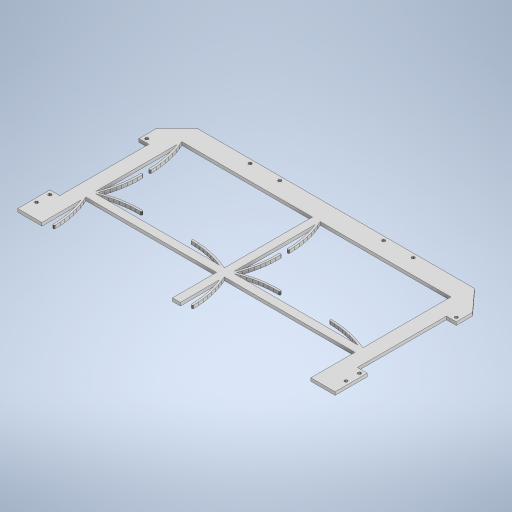
# Autodesk Inventor part: deck_top
Saved by Autodesk Inventor 2024.1 (Build 281209000, 209)
## iProperties
Created: 2024-06-24
Part Number: deck_top
Material: Generic
Document SubType Name: Modeling
Designer: pab2
Density: 1 g/cm^3
Appearance: Default
Author: pab2
Autodesk Inventor part; units mm, degrees
ref_plane "YZ Plane" through (0, 0, 0) normal (1, 0, 0) x (0, 1, 0)
ref_plane "XZ Plane" through (0, 0, 0) normal (0, 1, 0) x (-1, 0, 0)
ref_plane "XY Plane" through (0, 0, 0) normal (0, 0, 1) x (1, 0, 0)
sketch "Sketch1" plane through (0, 0, 0) normal (0, 1, 0) x (-1, 0, 0)
  line L0 (377.2253, 565.1147) -> (377.7897, 565.2558)
  line L1 (377.7897, 565.2558) -> (378.2836, 565.5733)
  line L2 (378.2836, 565.5733) -> (378.6011, 566.0672)
  line L3 (378.6011, 566.0672) -> (378.7422, 566.6316)
  line L4 (378.7422, 566.6316) -> (378.6011, 567.1961)
  line L5 (378.6011, 567.1961) -> (378.2836, 567.69)
  line L6 (378.2836, 567.69) -> (377.7897, 568.0075)
  line L7 (377.7897, 568.0075) -> (377.2253, 568.1133)
  line L8 (377.2253, 568.1133) -> (376.6608, 568.0075)
  line L9 (376.6608, 568.0075) -> (376.167, 567.69)
  line L10 (376.167, 567.69) -> (375.8495, 567.1961)
  line L11 (375.8495, 567.1961) -> (375.7436, 566.6316)
  line L12 (375.7436, 566.6316) -> (375.8495, 566.0672)
  line L13 (375.8495, 566.0672) -> (376.167, 565.5733)
  line L14 (376.167, 565.5733) -> (376.6608, 565.2558)
  line L15 (376.6608, 565.2558) -> (377.2253, 565.1147)
  line L16 (347.2392, 565.1147) -> (347.8036, 565.2558)
  line L17 (347.8036, 565.2558) -> (348.2975, 565.5733)
  line L18 (348.2975, 565.5733) -> (348.615, 566.0672)
  line L19 (348.615, 566.0672) -> (348.7208, 566.6316)
  line L20 (348.7208, 566.6316) -> (348.615, 567.1961)
  line L21 (348.615, 567.1961) -> (348.2975, 567.69)
  line L22 (348.2975, 567.69) -> (347.8036, 568.0075)
  line L23 (347.8036, 568.0075) -> (347.2392, 568.1133)
  line L24 (347.2392, 568.1133) -> (346.6395, 568.0075)
  line L25 (346.6395, 568.0075) -> (346.1809, 567.69)
  line L26 (346.1809, 567.69) -> (345.8281, 567.1961)
  line L27 (345.8281, 567.1961) -> (345.7222, 566.6316)
  line L28 (345.7222, 566.6316) -> (345.8281, 566.0672)
  line L29 (345.8281, 566.0672) -> (346.1809, 565.5733)
  line L30 (346.1809, 565.5733) -> (346.6395, 565.2558)
  line L31 (346.6395, 565.2558) -> (347.2392, 565.1147)
  line L32 (212.2311, 565.1147) -> (212.7956, 565.2558)
  line L33 (212.7956, 565.2558) -> (213.2895, 565.5733)
  line L34 (213.2895, 565.5733) -> (213.607, 566.0672)
  line L35 (213.607, 566.0672) -> (213.7128, 566.6316)
  line L36 (213.7128, 566.6316) -> (213.607, 567.1961)
  line L37 (213.607, 567.1961) -> (213.2895, 567.69)
  line L38 (213.2895, 567.69) -> (212.7956, 568.0075)
  line L39 (212.7956, 568.0075) -> (212.2311, 568.1133)
  line L40 (212.2311, 568.1133) -> (211.6667, 568.0075)
  line L41 (211.6667, 568.0075) -> (211.1728, 567.69)
  line L42 (211.1728, 567.69) -> (210.8553, 567.1961)
  line L43 (210.8553, 567.1961) -> (210.7142, 566.6316)
  line L44 (210.7142, 566.6316) -> (210.8553, 566.0672)
  line L45 (210.8553, 566.0672) -> (211.1728, 565.5733)
  line L46 (211.1728, 565.5733) -> (211.6667, 565.2558)
  line L47 (211.6667, 565.2558) -> (212.2311, 565.1147)
  line L48 (423.7214, 631.1547) -> (423.792, 635.9878)
  line L49 (423.792, 635.9878) -> (424.1094, 640.8208)
  line L50 (424.1094, 640.8208) -> (424.6386, 645.6186)
  line L51 (424.6386, 645.6186) -> (425.3795, 650.4164)
  line L52 (425.3795, 650.4164) -> (426.4025, 655.1436)
  line L53 (426.4025, 655.1436) -> (427.6019, 659.8356)
  line L54 (427.6019, 659.8356) -> (429.0483, 664.4569)
  line L55 (429.0483, 664.4569) -> (430.7417, 668.9725)
  line L56 (421.7106, 631.1194) -> (421.8164, 630.7314)
  line L57 (421.8164, 630.7314) -> (422.0281, 630.4139)
  line L58 (422.0281, 630.4139) -> (422.3455, 630.2022)
  line L59 (422.3455, 630.2022) -> (422.7336, 630.1316)
  line L60 (422.7336, 630.1316) -> (423.1217, 630.2022)
  line L61 (423.1217, 630.2022) -> (423.4392, 630.4139)
  line L62 (423.4392, 630.4139) -> (423.6508, 630.7667)
  line L63 (423.6508, 630.7667) -> (423.7214, 631.1547)
  line L64 (428.5897, 668.9725) -> (426.9316, 664.4217)
  line L65 (426.9316, 664.4217) -> (425.5205, 659.8003)
  line L66 (425.5205, 659.8003) -> (424.3211, 655.1083)
  line L67 (424.3211, 655.1083) -> (423.3686, 650.3811)
  line L68 (423.3686, 650.3811) -> (422.5925, 645.5833)
  line L69 (422.5925, 645.5833) -> (422.0986, 640.7856)
  line L70 (422.0986, 640.7856) -> (421.7811, 635.9525)
  line L71 (421.7811, 635.9525) -> (421.7106, 631.1194)
  line L72 (390.7014, 662.1286) -> (395.5697, 662.1992)
  line L73 (395.5697, 662.1992) -> (400.3675, 662.4814)
  line L74 (400.3675, 662.4814) -> (405.2005, 663.0106)
  line L75 (405.2005, 663.0106) -> (409.963, 663.7514)
  line L76 (409.963, 663.7514) -> (414.7255, 664.7391)
  line L77 (414.7255, 664.7391) -> (419.4175, 665.9386)
  line L78 (419.4175, 665.9386) -> (424.0389, 667.3497)
  line L79 (424.0389, 667.3497) -> (428.5897, 668.9725)
  line L80 (390.7367, 664.1394) -> (390.3486, 664.0689)
  line L81 (390.3486, 664.0689) -> (390.0311, 663.8572)
  line L82 (390.0311, 663.8572) -> (389.8194, 663.5397)
  line L83 (389.8194, 663.5397) -> (389.7136, 663.1516)
  line L84 (389.7136, 663.1516) -> (389.7842, 662.7636)
  line L85 (389.7842, 662.7636) -> (389.9958, 662.4461)
  line L86 (389.9958, 662.4461) -> (390.3486, 662.1992)
  line L87 (390.3486, 662.1992) -> (390.7014, 662.1286)
  line L88 (428.5897, 671.1245) -> (424.0389, 669.4664)
  line L89 (424.0389, 669.4664) -> (419.4175, 668.02)
  line L90 (419.4175, 668.02) -> (414.7255, 666.7853)
  line L91 (414.7255, 666.7853) -> (409.9983, 665.7975)
  line L92 (409.9983, 665.7975) -> (405.2358, 665.0214)
  line L93 (405.2358, 665.0214) -> (400.4028, 664.4922)
  line L94 (400.4028, 664.4922) -> (395.5697, 664.21)
  line L95 (395.5697, 664.21) -> (390.7367, 664.1394)
  line L96 (428.5897, 671.1245) -> (303.8475, 671.1245)
  line L97 (338.7372, 664.1394) -> (334.2922, 664.3158)
  line L98 (334.2922, 664.3158) -> (329.812, 664.7039)
  line L99 (329.812, 664.7039) -> (325.4022, 665.2683)
  line L100 (325.4022, 665.2683) -> (320.9925, 666.0797)
  line L101 (320.9925, 666.0797) -> (316.6181, 667.0322)
  line L102 (316.6181, 667.0322) -> (312.3142, 668.2316)
  line L103 (312.3142, 668.2316) -> (308.0456, 669.5722)
  line L104 (308.0456, 669.5722) -> (303.8475, 671.1245)
  line L105 (338.702, 662.1286) -> (339.09, 662.1992)
  line L106 (339.09, 662.1992) -> (339.4075, 662.4108)
  line L107 (339.4075, 662.4108) -> (339.6545, 662.7283)
  line L108 (339.6545, 662.7283) -> (339.725, 663.1164)
  line L109 (339.725, 663.1164) -> (339.6545, 663.5044)
  line L110 (339.6545, 663.5044) -> (339.4428, 663.8219)
  line L111 (339.4428, 663.8219) -> (339.1253, 664.0336)
  line L112 (339.1253, 664.0336) -> (338.7372, 664.1394)
  line L113 (298.7322, 671.1245) -> (303.4947, 669.1136)
  line L114 (303.4947, 669.1136) -> (308.3278, 667.385)
  line L115 (308.3278, 667.385) -> (313.2667, 665.8681)
  line L116 (313.2667, 665.8681) -> (318.2761, 664.5981)
  line L117 (318.2761, 664.5981) -> (323.3208, 663.6103)
  line L118 (323.3208, 663.6103) -> (328.4361, 662.8342)
  line L119 (328.4361, 662.8342) -> (333.5514, 662.3755)
  line L120 (333.5514, 662.3755) -> (338.702, 662.1286)
  line L121 (298.7322, 671.1245) -> (298.7322, 582.1186)
  line L122 (298.7322, 582.1186) -> (430.7417, 582.1186)
  line L123 (421.7106, 622.1236) -> (421.9575, 616.9731)
  line L124 (421.9575, 616.9731) -> (422.4514, 611.8225)
  line L125 (422.4514, 611.8225) -> (423.1922, 606.7072)
  line L126 (423.1922, 606.7072) -> (424.2153, 601.6625)
  line L127 (424.2153, 601.6625) -> (425.45, 596.653)
  line L128 (425.45, 596.653) -> (426.967, 591.7141)
  line L129 (426.967, 591.7141) -> (428.7309, 586.8811)
  line L130 (428.7309, 586.8811) -> (430.7417, 582.1186)
  line L131 (423.7214, 622.1589) -> (423.6508, 622.5469)
  line L132 (423.6508, 622.5469) -> (423.4039, 622.8644)
  line L133 (423.4039, 622.8644) -> (423.0864, 623.0761)
  line L134 (423.0864, 623.0761) -> (422.6983, 623.1467)
  line L135 (422.6983, 623.1467) -> (422.3103, 623.0408)
  line L136 (422.3103, 623.0408) -> (421.9928, 622.8292)
  line L137 (421.9928, 622.8292) -> (421.7811, 622.5117)
  line L138 (421.7811, 622.5117) -> (421.7106, 622.1236)
  line L139 (430.7417, 587.2691) -> (429.1894, 591.4672)
  line L140 (429.1894, 591.4672) -> (427.8136, 595.7005)
  line L141 (427.8136, 595.7005) -> (426.6495, 600.0397)
  line L142 (426.6495, 600.0397) -> (425.6617, 604.3789)
  line L143 (425.6617, 604.3789) -> (424.8856, 608.7886)
  line L144 (424.8856, 608.7886) -> (424.2858, 613.2336)
  line L145 (424.2858, 613.2336) -> (423.8978, 617.6786)
  line L146 (423.8978, 617.6786) -> (423.7214, 622.1589)
  line L147 (430.7417, 587.2691) -> (430.7417, 668.9725)
  line L148 (281.7283, 622.1236) -> (281.94, 616.9731)
  line L149 (281.94, 616.9731) -> (282.4339, 611.8225)
  line L150 (282.4339, 611.8225) -> (283.21, 606.7072)
  line L151 (283.21, 606.7072) -> (284.1978, 601.6625)
  line L152 (284.1978, 601.6625) -> (285.4678, 596.653)
  line L153 (285.4678, 596.653) -> (286.9847, 591.7141)
  line L154 (286.9847, 591.7141) -> (288.7133, 586.8811)
  line L155 (288.7133, 586.8811) -> (290.7242, 582.1186)
  line L156 (283.7392, 622.1589) -> (283.6334, 622.5469)
  line L157 (283.6334, 622.5469) -> (283.4217, 622.8644)
  line L158 (283.4217, 622.8644) -> (283.1042, 623.0761)
  line L159 (283.1042, 623.0761) -> (282.7161, 623.1467)
  line L160 (282.7161, 623.1467) -> (282.3281, 623.0408)
  line L161 (282.3281, 623.0408) -> (282.0106, 622.8292)
  line L162 (282.0106, 622.8292) -> (281.7989, 622.5117)
  line L163 (281.7989, 622.5117) -> (281.7283, 622.1236)
  line L164 (290.7242, 587.2691) -> (289.1719, 591.4672)
  line L165 (289.1719, 591.4672) -> (287.7961, 595.7005)
  line L166 (287.7961, 595.7005) -> (286.632, 600.0397)
  line L167 (286.632, 600.0397) -> (285.6795, 604.3789)
  line L168 (285.6795, 604.3789) -> (284.8681, 608.7886)
  line L169 (284.8681, 608.7886) -> (284.3036, 613.2336)
  line L170 (284.3036, 613.2336) -> (283.9156, 617.6786)
  line L171 (283.9156, 617.6786) -> (283.7392, 622.1589)
  line L172 (290.7242, 587.2691) -> (290.7242, 668.9725)
  line L173 (283.7392, 631.1547) -> (283.8097, 635.9878)
  line L174 (283.8097, 635.9878) -> (284.092, 640.8208)
  line L175 (284.092, 640.8208) -> (284.6211, 645.6186)
  line L176 (284.6211, 645.6186) -> (285.3972, 650.4164)
  line L177 (285.3972, 650.4164) -> (286.385, 655.1436)
  line L178 (286.385, 655.1436) -> (287.6197, 659.8356)
  line L179 (287.6197, 659.8356) -> (289.0661, 664.4569)
  line L180 (289.0661, 664.4569) -> (290.7242, 668.9725)
  line L181 (281.7283, 631.1194) -> (281.7989, 630.7314)
  line L182 (281.7989, 630.7314) -> (282.0106, 630.4139)
  line L183 (282.0106, 630.4139) -> (282.3633, 630.2022)
  line L184 (282.3633, 630.2022) -> (282.7514, 630.1316)
  line L185 (282.7514, 630.1316) -> (283.1042, 630.2022)
  line L186 (283.1042, 630.2022) -> (283.457, 630.4139)
  line L187 (283.457, 630.4139) -> (283.6686, 630.7667)
  line L188 (283.6686, 630.7667) -> (283.7392, 631.1547)
  line L189 (288.5722, 668.9725) -> (286.9495, 664.4217)
  line L190 (286.9495, 664.4217) -> (285.5383, 659.8003)
  line L191 (285.5383, 659.8003) -> (284.3389, 655.1083)
  line L192 (284.3389, 655.1083) -> (283.3511, 650.3811)
  line L193 (283.3511, 650.3811) -> (282.6103, 645.5833)
  line L194 (282.6103, 645.5833) -> (282.0811, 640.7856)
  line L195 (282.0811, 640.7856) -> (281.7989, 635.9525)
  line L196 (281.7989, 635.9525) -> (281.7283, 631.1194)
  line L197 (250.7192, 662.1286) -> (255.5522, 662.1992)
  line L198 (255.5522, 662.1992) -> (260.3853, 662.4814)
  line L199 (260.3853, 662.4814) -> (265.1831, 663.0106)
  line L200 (265.1831, 663.0106) -> (269.9809, 663.7514)
  line L201 (269.9809, 663.7514) -> (274.7081, 664.7391)
  line L202 (274.7081, 664.7391) -> (279.4, 665.9386)
  line L203 (279.4, 665.9386) -> (284.0214, 667.3497)
  line L204 (284.0214, 667.3497) -> (288.5722, 668.9725)
  line L205 (250.7545, 664.1394) -> (250.3664, 664.0689)
  line L206 (250.3664, 664.0689) -> (250.0136, 663.8572)
  line L207 (250.0136, 663.8572) -> (249.802, 663.5397)
  line L208 (249.802, 663.5397) -> (249.7314, 663.1516)
  line L209 (249.7314, 663.1516) -> (249.802, 662.7636)
  line L210 (249.802, 662.7636) -> (250.0136, 662.4461)
  line L211 (250.0136, 662.4461) -> (250.3311, 662.1992)
  line L212 (250.3311, 662.1992) -> (250.7192, 662.1286)
  line L213 (288.5722, 671.1245) -> (284.0214, 669.4664)
  line L214 (284.0214, 669.4664) -> (279.4353, 668.02)
  line L215 (279.4353, 668.02) -> (274.7434, 666.7853)
  line L216 (274.7434, 666.7853) -> (270.0161, 665.7975)
  line L217 (270.0161, 665.7975) -> (265.2184, 665.0214)
  line L218 (265.2184, 665.0214) -> (260.4206, 664.4922)
  line L219 (260.4206, 664.4922) -> (255.5875, 664.21)
  line L220 (255.5875, 664.21) -> (250.7545, 664.1394)
  line L221 (288.5722, 671.1245) -> (163.8653, 671.1245)
  line L222 (198.755, 664.1394) -> (194.2747, 664.3158)
  line L223 (194.2747, 664.3158) -> (189.8297, 664.7039)
  line L224 (189.8297, 664.7039) -> (185.3847, 665.2683)
  line L225 (185.3847, 665.2683) -> (180.975, 666.0797)
  line L226 (180.975, 666.0797) -> (176.6359, 667.0322)
  line L227 (176.6359, 667.0322) -> (172.2967, 668.2316)
  line L228 (172.2967, 668.2316) -> (168.0633, 669.5722)
  line L229 (168.0633, 669.5722) -> (163.8653, 671.1245)
  line L230 (198.7197, 662.1286) -> (199.1078, 662.1992)
  line L231 (199.1078, 662.1992) -> (199.4253, 662.4108)
  line L232 (199.4253, 662.4108) -> (199.637, 662.7283)
  line L233 (199.637, 662.7283) -> (199.7428, 663.1164)
  line L234 (199.7428, 663.1164) -> (199.6722, 663.5044)
  line L235 (199.6722, 663.5044) -> (199.4606, 663.8219)
  line L236 (199.4606, 663.8219) -> (199.1431, 664.0336)
  line L237 (199.1431, 664.0336) -> (198.755, 664.1394)
  line L238 (158.7147, 671.1245) -> (163.4772, 669.1136)
  line L239 (163.4772, 669.1136) -> (168.3456, 667.385)
  line L240 (168.3456, 667.385) -> (173.2492, 665.8681)
  line L241 (173.2492, 665.8681) -> (178.2586, 664.5981)
  line L242 (178.2586, 664.5981) -> (183.3033, 663.6103)
  line L243 (183.3033, 663.6103) -> (188.4186, 662.8342)
  line L244 (188.4186, 662.8342) -> (193.5692, 662.3755)
  line L245 (193.5692, 662.3755) -> (198.7197, 662.1286)
  line L246 (158.7147, 671.1245) -> (158.7147, 582.1186)
  line L247 (158.7147, 582.1186) -> (290.7242, 582.1186)
  line L248 (451.238, 707.1431) -> (451.8025, 707.2489)
  line L249 (451.8025, 707.2489) -> (452.2964, 707.5664)
  line L250 (452.2964, 707.5664) -> (452.6139, 708.0603)
  line L251 (452.6139, 708.0603) -> (452.7197, 708.6247)
  line L252 (452.7197, 708.6247) -> (452.6139, 709.1891)
  line L253 (452.6139, 709.1891) -> (452.2964, 709.683)
  line L254 (452.2964, 709.683) -> (451.8025, 710.0005)
  line L255 (451.8025, 710.0005) -> (451.238, 710.1417)
  line L256 (451.238, 710.1417) -> (450.6383, 710.0005)
  line L257 (450.6383, 710.0005) -> (450.1797, 709.683)
  line L258 (450.1797, 709.683) -> (449.8269, 709.1891)
  line L259 (449.8269, 709.1891) -> (449.7211, 708.6247)
  line L260 (449.7211, 708.6247) -> (449.8269, 708.0603)
  line L261 (449.8269, 708.0603) -> (450.1797, 707.5664)
  line L262 (450.1797, 707.5664) -> (450.6383, 707.2489)
  line L263 (450.6383, 707.2489) -> (451.238, 707.1431)
  line L264 (242.2172, 565.1147) -> (242.817, 565.2558)
  line L265 (242.817, 565.2558) -> (243.2756, 565.5733)
  line L266 (243.2756, 565.5733) -> (243.6283, 566.0672)
  line L267 (243.6283, 566.0672) -> (243.7342, 566.6316)
  line L268 (243.7342, 566.6316) -> (243.6283, 567.1961)
  line L269 (243.6283, 567.1961) -> (243.2756, 567.69)
  line L270 (243.2756, 567.69) -> (242.817, 568.0075)
  line L271 (242.817, 568.0075) -> (242.2172, 568.1133)
  line L272 (242.2172, 568.1133) -> (241.6528, 568.0075)
  line L273 (241.6528, 568.0075) -> (241.1589, 567.69)
  line L274 (241.1589, 567.69) -> (240.8414, 567.1961)
  line L275 (240.8414, 567.1961) -> (240.7356, 566.6316)
  line L276 (240.7356, 566.6316) -> (240.8414, 566.0672)
  line L277 (240.8414, 566.0672) -> (241.1589, 565.5733)
  line L278 (241.1589, 565.5733) -> (241.6528, 565.2558)
  line L279 (241.6528, 565.2558) -> (242.2172, 565.1147)
  line L280 (138.2184, 707.1431) -> (138.8181, 707.2489)
  line L281 (138.8181, 707.2489) -> (139.2767, 707.5664)
  line L282 (139.2767, 707.5664) -> (139.6295, 708.0603)
  line L283 (139.6295, 708.0603) -> (139.7353, 708.6247)
  line L284 (139.7353, 708.6247) -> (139.6295, 709.1891)
  line L285 (139.6295, 709.1891) -> (139.2767, 709.683)
  line L286 (139.2767, 709.683) -> (138.8181, 710.0005)
  line L287 (138.8181, 710.0005) -> (138.2184, 710.1417)
  line L288 (138.2184, 710.1417) -> (137.6539, 710.0005)
  line L289 (137.6539, 710.0005) -> (137.16, 709.683)
  line L290 (137.16, 709.683) -> (136.8425, 709.1891)
  line L291 (136.8425, 709.1891) -> (136.7367, 708.6247)
  line L292 (136.7367, 708.6247) -> (136.8425, 708.0603)
  line L293 (136.8425, 708.0603) -> (137.16, 707.5664)
  line L294 (137.16, 707.5664) -> (137.6539, 707.2489)
  line L295 (137.6539, 707.2489) -> (138.2184, 707.1431)
  line L296 (138.2184, 595.5947) -> (138.8181, 595.7005)
  line L297 (138.8181, 595.7005) -> (139.2767, 596.0181)
  line L298 (139.2767, 596.0181) -> (139.6295, 596.512)
  line L299 (139.6295, 596.512) -> (139.7353, 597.0764)
  line L300 (139.7353, 597.0764) -> (139.6295, 597.6761)
  line L301 (139.6295, 597.6761) -> (139.2767, 598.1347)
  line L302 (139.2767, 598.1347) -> (138.8181, 598.4875)
  line L303 (138.8181, 598.4875) -> (138.2184, 598.5933)
  line L304 (138.2184, 598.5933) -> (137.6539, 598.4875)
  line L305 (137.6539, 598.4875) -> (137.16, 598.1347)
  line L306 (137.16, 598.1347) -> (136.8425, 597.6761)
  line L307 (136.8425, 597.6761) -> (136.7367, 597.0764)
  line L308 (136.7367, 597.0764) -> (136.8425, 596.512)
  line L309 (136.8425, 596.512) -> (137.16, 596.0181)
  line L310 (137.16, 596.0181) -> (137.6539, 595.7005)
  line L311 (137.6539, 595.7005) -> (138.2184, 595.5947)
  line L312 (434.2342, 562.6453) -> (455.2245, 583.6356)
  line L313 (154.2345, 562.6453) -> (434.2342, 562.6453)
  line L314 (134.232, 584.588) -> (154.2345, 562.6453)
  line L315 (134.232, 601.0981) -> (134.232, 584.588)
  line L316 (134.232, 601.0981) -> (144.2156, 601.0981)
  line L317 (144.2156, 601.0981) -> (144.2156, 691.0917)
  line L318 (144.2156, 691.0917) -> (134.232, 691.0917)
  line L319 (158.7147, 723.6178) -> (134.232, 723.6178)
  line L320 (158.7147, 679.1325) -> (158.7147, 723.6178)
  line L321 (290.7242, 679.1325) -> (158.7147, 679.1325)
  line L322 (281.7283, 719.1022) -> (281.94, 713.9516)
  line L323 (281.94, 713.9516) -> (282.4339, 708.8364)
  line L324 (282.4339, 708.8364) -> (283.21, 703.7211)
  line L325 (283.21, 703.7211) -> (284.1978, 698.6764)
  line L326 (284.1978, 698.6764) -> (285.4678, 693.6669)
  line L327 (285.4678, 693.6669) -> (286.9847, 688.728)
  line L328 (286.9847, 688.728) -> (288.7133, 683.895)
  line L329 (288.7133, 683.895) -> (290.7242, 679.1325)
  line L330 (283.7392, 719.1375) -> (283.6334, 719.5255)
  line L331 (283.6334, 719.5255) -> (283.4217, 719.8431)
  line L332 (283.4217, 719.8431) -> (283.1042, 720.0547)
  line L333 (283.1042, 720.0547) -> (282.7161, 720.1253)
  line L334 (282.7161, 720.1253) -> (282.3281, 720.0547)
  line L335 (282.3281, 720.0547) -> (282.0106, 719.8078)
  line L336 (282.0106, 719.8078) -> (281.7989, 719.4903)
  line L337 (281.7989, 719.4903) -> (281.7283, 719.1022)
  line L338 (290.7242, 684.2478) -> (289.1719, 688.4458)
  line L339 (289.1719, 688.4458) -> (287.7961, 692.7144)
  line L340 (287.7961, 692.7144) -> (286.632, 697.0183)
  line L341 (286.632, 697.0183) -> (285.6795, 701.3928)
  line L342 (285.6795, 701.3928) -> (284.8681, 705.8025)
  line L343 (284.8681, 705.8025) -> (284.3036, 710.2122)
  line L344 (284.3036, 710.2122) -> (283.9156, 714.6925)
  line L345 (283.9156, 714.6925) -> (283.7392, 719.1375)
  line L346 (290.7242, 723.6178) -> (290.7242, 684.2478)
  line L347 (298.7322, 723.6178) -> (290.7242, 723.6178)
  line L348 (298.7322, 679.1325) -> (298.7322, 723.6178)
  line L349 (430.7417, 679.1325) -> (298.7322, 679.1325)
  line L350 (421.7106, 719.1022) -> (421.9575, 713.9516)
  line L351 (421.9575, 713.9516) -> (422.4514, 708.8364)
  line L352 (422.4514, 708.8364) -> (423.1922, 703.7211)
  line L353 (423.1922, 703.7211) -> (424.2153, 698.6764)
  line L354 (424.2153, 698.6764) -> (425.45, 693.6669)
  line L355 (425.45, 693.6669) -> (426.967, 688.728)
  line L356 (426.967, 688.728) -> (428.7309, 683.895)
  line L357 (428.7309, 683.895) -> (430.7417, 679.1325)
  line L358 (423.7214, 719.1375) -> (423.6508, 719.5255)
  line L359 (423.6508, 719.5255) -> (423.4039, 719.8431)
  line L360 (423.4039, 719.8431) -> (423.0864, 720.0547)
  line L361 (423.0864, 720.0547) -> (422.6983, 720.1253)
  line L362 (422.6983, 720.1253) -> (422.3103, 720.0547)
  line L363 (422.3103, 720.0547) -> (421.9928, 719.8078)
  line L364 (421.9928, 719.8078) -> (421.7811, 719.4903)
  line L365 (421.7811, 719.4903) -> (421.7106, 719.1022)
  line L366 (430.7417, 684.2478) -> (429.1894, 688.4458)
  line L367 (429.1894, 688.4458) -> (427.8136, 692.7144)
  line L368 (427.8136, 692.7144) -> (426.6495, 697.0183)
  line L369 (426.6495, 697.0183) -> (425.6617, 701.3928)
  line L370 (425.6617, 701.3928) -> (424.8856, 705.8025)
  line L371 (424.8856, 705.8025) -> (424.2858, 710.2122)
  line L372 (424.2858, 710.2122) -> (423.8978, 714.6925)
  line L373 (423.8978, 714.6925) -> (423.7214, 719.1375)
  line L374 (430.7417, 723.6178) -> (430.7417, 684.2478)
  line L375 (455.2245, 723.6178) -> (430.7417, 723.6178)
  line L376 (455.2245, 691.0917) -> (455.2245, 723.6178)
  line L377 (455.2245, 691.0917) -> (445.2408, 691.0917)
  line L378 (445.2408, 691.0917) -> (445.2408, 601.0981)
  line L379 (445.2408, 601.0981) -> (455.2245, 601.0981)
  line L380 (138.2184, 693.5964) -> (138.8181, 693.7022)
  line L381 (138.8181, 693.7022) -> (139.2767, 694.0197)
  line L382 (139.2767, 694.0197) -> (139.6295, 694.5136)
  line L383 (139.6295, 694.5136) -> (139.7353, 695.078)
  line L384 (139.7353, 695.078) -> (139.6295, 695.6425)
  line L385 (139.6295, 695.6425) -> (139.2767, 696.1364)
  line L386 (139.2767, 696.1364) -> (138.8181, 696.4539)
  line L387 (138.8181, 696.4539) -> (138.2184, 696.595)
  line L388 (138.2184, 696.595) -> (137.6539, 696.4539)
  line L389 (137.6539, 696.4539) -> (137.16, 696.1364)
  line L390 (137.16, 696.1364) -> (136.8425, 695.6425)
  line L391 (136.8425, 695.6425) -> (136.7367, 695.078)
  line L392 (136.7367, 695.078) -> (136.8425, 694.5136)
  line L393 (136.8425, 694.5136) -> (137.16, 694.0197)
  line L394 (137.16, 694.0197) -> (137.6539, 693.7022)
  line L395 (137.6539, 693.7022) -> (138.2184, 693.5964)
  line L396 (451.238, 693.5964) -> (451.8025, 693.7022)
  line L397 (451.8025, 693.7022) -> (452.2964, 694.0197)
  line L398 (452.2964, 694.0197) -> (452.6139, 694.5136)
  line L399 (452.6139, 694.5136) -> (452.7197, 695.078)
  line L400 (452.7197, 695.078) -> (452.6139, 695.6425)
  line L401 (452.6139, 695.6425) -> (452.2964, 696.1364)
  line L402 (452.2964, 696.1364) -> (451.8025, 696.4539)
  line L403 (451.8025, 696.4539) -> (451.238, 696.595)
  line L404 (451.238, 696.595) -> (450.6383, 696.4539)
  line L405 (450.6383, 696.4539) -> (450.1797, 696.1364)
  line L406 (450.1797, 696.1364) -> (449.8269, 695.6425)
  line L407 (449.8269, 695.6425) -> (449.7211, 695.078)
  line L408 (449.7211, 695.078) -> (449.8269, 694.5136)
  line L409 (449.8269, 694.5136) -> (450.1797, 694.0197)
  line L410 (450.1797, 694.0197) -> (450.6383, 693.7022)
  line L411 (450.6383, 693.7022) -> (451.238, 693.5964)
  line L412 (451.238, 595.5947) -> (451.8025, 595.7005)
  line L413 (451.8025, 595.7005) -> (452.2964, 596.0181)
  line L414 (452.2964, 596.0181) -> (452.6139, 596.512)
  line L415 (452.6139, 596.512) -> (452.7197, 597.0764)
  line L416 (452.7197, 597.0764) -> (452.6139, 597.6761)
  line L417 (452.6139, 597.6761) -> (452.2964, 598.1347)
  line L418 (452.2964, 598.1347) -> (451.8025, 598.4875)
  line L419 (451.8025, 598.4875) -> (451.238, 598.5933)
  line L420 (451.238, 598.5933) -> (450.6383, 598.4875)
  line L421 (450.6383, 598.4875) -> (450.1797, 598.1347)
  line L422 (450.1797, 598.1347) -> (449.8269, 597.6761)
  line L423 (449.8269, 597.6761) -> (449.7211, 597.0764)
  line L424 (449.7211, 597.0764) -> (449.8269, 596.512)
  line L425 (449.8269, 596.512) -> (450.1797, 596.0181)
  line L426 (450.1797, 596.0181) -> (450.6383, 595.7005)
  line L427 (450.6383, 595.7005) -> (451.238, 595.5947)
  line L428 (455.2245, 583.6356) -> (455.2245, 601.0981)
  line L429 (134.232, 723.6178) -> (134.232, 691.0917)
  point P0 (0, 0)
  constraints: 860 end point
extrude "Extrusion1" add sketch "Sketch1" along normal blind 3.175
body "Solid1"
